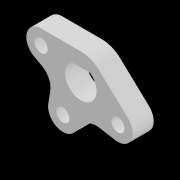
# Autodesk Inventor part: ShaftLock
Saved by Autodesk Inventor 2020 (Build 240168000, 168)
## iProperties
Created: 2021-01-24
Part Number: ShaftLock
Material: Generic
Document SubType Name: Sheet Metal
Designer: valer
Density: 1 g/cm^3
Sheet Metal Rule: Default
Appearance: Default
Author: valer
Autodesk Inventor part; units mm, degrees
ref_plane "YZ Plane" through (0, 0, 0) normal (1, 0, 0) x (0, 1, 0)
ref_plane "XZ Plane" through (0, 0, 0) normal (0, 1, 0) x (-1, 0, 0)
ref_plane "XY Plane" through (0, 0, 0) normal (0, 0, 1) x (1, 0, 0)
sketch "Sketch2" plane through (0, 0, 0) normal (0, 0, 1) x (1, 0, 0)
  circle A0 centre (46.408, 50.5954) radius 3.175 construction
  circle A1 centre (46.408, 50.5954) radius 5.08
  line L0 (46.408, 50.5954) -> (38.8405, 52.8571) construction
  line L1 (46.408, 50.5954) -> (53.477, 47.0722) construction
  circle A2 centre (38.8405, 52.8571) radius 2.8183
  circle A3 centre (53.477, 47.0722) radius 2.8183
  circle A4 centre (38.8405, 52.8571) radius 1.25
  circle A5 centre (53.477, 47.0722) radius 1.25
  line L2 (38.8405, 55.6754) -> (46.408, 55.6754)
  line L3 (37.5063, 50.3746) -> (42.0976, 47.9072)
  line L4 (55.4024, 49.1303) -> (50.0414, 54.1458)
  line L5 (52.3888, 44.4725) -> (48.6507, 46.0372)
  circle A6 centre (46.408, 50.5954) radius 3
  circle A7 centre (46.408, 50.5954) radius 4.2333 construction
  line L6 (46.408, 50.5954) -> (42.9902, 43.4749) construction
  circle A8 centre (42.9902, 43.4749) radius 1.25
  circle A9 centre (42.9902, 43.4749) radius 2.8183
  line L7 (40.2199, 43.993) -> (41.3557, 50.0663)
  line L8 (45.2023, 41.7287) -> (48.5744, 46.0005)
  point P0 (0, 0)
  dimension "d7" = 10.16
  dimension "d8" = 2.5
  dimension "d9" = 6
  dimension "d10" = 8.4667
  measures "d7" diameter of A1
  measures "d8" diameter of A4
  measures "d9" diameter of A6
  measures "d10" diameter of A7
extrude "Plate2" add sketch "Sketch2" along normal blind 4 contours A1 | A3 | A1 A2 L2 | A1 L7 L3 A2 | A2 | A1 L3 L7 | A9
sketch "Sketch3" plane through (0, 0, 4) normal (0, 0, 1) x (1, 0, 0)
  arc A0 (42.0976, 47.9072) -> (44.2097, 46.0157) centre (46.408, 50.5954) ccw
  circle A1 centre (46.408, 50.5954) radius 5.08
  circle A2 centre (42.9902, 43.4749) radius 2.8183
  line L0 (40.2108, 43.9416) -> (41.328, 50.5954)
  line L1 (45.1528, 41.6677) -> (48.9266, 46.1837)
  arc A3 (44.2097, 46.0157) -> (50.9546, 48.3294) centre (46.408, 50.5954) ccw
  point P0 (0, 0)
sheet face with bend "Face3" sketch "Sketch3" thickness 4 toward (0, 0, -1) bend radius 4 contours A0 A2 L0 A1 | A1 L1 A2
bend "Bend1"
sketch "Sketch4" plane through (0, 0, 4) normal (0, 0, 1) x (1, 0, 0)
  arc A0 (50.9546, 48.3294) -> (46.408, 55.6754) centre (46.408, 50.5954) ccw
  arc A1 (50.9546, 48.3294) -> (46.408, 55.6754) centre (46.408, 50.5954) ccw
  circle A2 centre (46.408, 50.5954) radius 5.08
  circle A3 centre (53.477, 47.0722) radius 2.8183
  line L0 (55.4038, 49.129) -> (49.8811, 54.3027)
  line L1 (52.9948, 44.2955) -> (45.5388, 45.5903)
  arc A4 (44.2097, 46.0157) -> (50.9546, 48.3294) centre (46.408, 50.5954) ccw
  line L2 (49.8811, 54.3027) -> (45.5388, 45.5903)
  point P0 (0, 0)
sheet face with bend "Face4" sketch "Sketch4" thickness 4 toward (0, 0, -1) bend radius 4 picked at (48.6605, 51.1377) contours A2 L2 A0 | A3 L1 A2 | A0 L0 A3
bend "Bend2"
sketch "Sketch5" plane through (0, 0, 4) normal (0, 0, 1) x (1, 0, 0)
  arc A0 (48.8803, 52.2948) -> (46.5396, 47.5983) centre (46.408, 50.5954) ccw projected
  arc A1 (48.8803, 52.2948) -> (46.5396, 47.5983) centre (46.408, 50.5954) ccw projected
  circle A2 centre (46.408, 50.5954) radius 3
  point P0 (0, 0)
  point P1 (46.5396, 47.5983)
  constraints: 1 coincident, 3 other
extrude "Extrusion1" cut sketch "Sketch5" against normal blind 25.4
fillet "Fillet1" radius 3.175 2 edges at (40.9777, 48.509, 2) (48.0642, 45.1518, 2)
sketch "Sketch6" plane through (0, 0, 4) normal (0, 0, 1) x (1, 0, 0)
  circle A0 centre (46.408, 50.5954) radius 3 projected
  line L0 (43.408, 53.5954) -> (49.408, 53.5954)
  line L1 (49.408, 53.5954) -> (49.408, 47.5954)
  line L2 (49.408, 47.5954) -> (43.408, 47.5954)
  line L3 (43.408, 47.5954) -> (43.408, 53.5954)
  line L4 (43.408, 52.9954) -> (49.408, 52.9954)
  point P0 (0, 0)
  point P1 (44.608, 52.9954)
  point P2 (48.208, 52.9954)
  dimension "d26" = 5.4
  constraints: 10 end point, 4 tangent, 2 parallel, 2 perpendicular, 2 point on line, 1 horizontal
  measures "d26" distance between parallel lines of L2 L4
extrude "Extrusion2" add sketch "Sketch6" against normal up to surface (4 mm away) contours L4 A0 picked at (46.6209, 53.1725)
equation "\"d12\" = Thickness"
equation "\"d13\" = BendRadius"
equation "\"d14\" = BendReliefWidth"
equation "\"d16\" = MinimumRemnant"
equation "\"d15\" = BendReliefDepth"
equation "\"d17\" = TransitionRadius"
equation "\"d18\" = BendRadius"
equation "\"d19\" = BendReliefWidth"
equation "\"d21\" = MinimumRemnant"
equation "\"d20\" = BendReliefDepth"
equation "\"d22\" = TransitionRadius"
equation "\"BendRadius\" = Thickness"
equation "\"BendReliefWidth\" = Thickness"
equation "\"BendReliefDepth\" = 0.5 * Thickness"
equation "\"CornerReliefSize\" = 4 * Thickness"
equation "\"MinimumRemnant\" = 2 * Thickness"
equation "\"TransitionRadius\" = BendRadius"
equation "\"JacobiRadiusSize\" = BendRadius"
equation "\"GapSize\" = Thickness"
equation "\"Thickness\" = 4"
body "Solid2"
